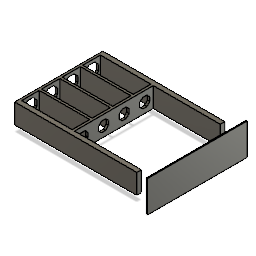
Toolkit Stand v3 (Autodesk Fusion 360 design; units mm, degrees)
Autodesk Fusion 360 part; units mm, degrees
sketch "Sketch1" plane through (0, 0, 0) normal (1, 0, 0) x (0, 0, -1)
  line L0 (0, 0) -> (75, 0)
  line L1 (75, 0) -> (75, 13)
  line L2 (75, 13) -> (0, 13)
  line L3 (0, 13) -> (0, 0)
  line L4 (37.5, 0) -> (37.5, 13)
  line L5 (37.5, 6.5) -> (34.5, 6.5)
  line L6 (37.5, 6.5) -> (40.5, 6.5)
  line L7 (34.5, 6.5) -> (23, 6.5)
  line L8 (34.5, 8.8817) -> (31.1317, 12.25)
  line L9 (31.1317, 12.25) -> (26.3683, 12.25)
  line L10 (26.3683, 12.25) -> (23, 8.8817)
  line L11 (23, 8.8817) -> (23, 4.1183)
  line L12 (23, 4.1183) -> (26.3683, 0.75)
  line L13 (26.3683, 0.75) -> (31.1317, 0.75)
  line L14 (31.1317, 0.75) -> (34.5, 4.1183)
  line L15 (34.5, 4.1183) -> (34.5, 8.8817)
  line L16 (23, 6.5) -> (17, 6.5)
  line L17 (17, 6.5) -> (5.5, 6.5)
  line L18 (5.5, 4.1183) -> (8.8683, 0.75)
  line L19 (8.8683, 0.75) -> (13.6317, 0.75)
  line L20 (13.6317, 0.75) -> (17, 4.1183)
  line L21 (17, 4.1183) -> (17, 8.8817)
  line L22 (17, 8.8817) -> (13.6317, 12.25)
  line L23 (13.6317, 12.25) -> (8.8683, 12.25)
  line L24 (8.8683, 12.25) -> (5.5, 8.8817)
  line L25 (5.5, 8.8817) -> (5.5, 4.1183)
  line L26 (40.5, 6.5) -> (52, 6.5)
  line L27 (40.5, 4.1183) -> (43.8683, 0.75)
  line L28 (43.8683, 0.75) -> (48.6317, 0.75)
  line L29 (48.6317, 0.75) -> (52, 4.1183)
  line L30 (52, 4.1183) -> (52, 8.8817)
  line L31 (52, 8.8817) -> (48.6317, 12.25)
  line L32 (48.6317, 12.25) -> (43.8683, 12.25)
  line L33 (43.8683, 12.25) -> (40.5, 8.8817)
  line L34 (40.5, 8.8817) -> (40.5, 4.1183)
  line L35 (52, 6.5) -> (58, 6.5)
  line L36 (58, 6.5) -> (69.5, 6.5)
  line L37 (58, 4.1183) -> (61.3683, 0.75)
  line L38 (61.3683, 0.75) -> (66.1317, 0.75)
  line L39 (66.1317, 0.75) -> (69.5, 4.1183)
  line L40 (69.5, 4.1183) -> (69.5, 8.8817)
  line L41 (69.5, 8.8817) -> (66.1317, 12.25)
  line L42 (66.1317, 12.25) -> (61.3683, 12.25)
  line L43 (61.3683, 12.25) -> (58, 8.8817)
  line L44 (58, 8.8817) -> (58, 4.1183)
  point P0 (28.75, 6.5)
  point P1 (11.25, 6.5)
  point P2 (46.25, 6.5)
  point P3 (63.75, 6.5)
  dimension "d1" = 75
  dimension "d2" = 13
  dimension "d3" = 3
  dimension "d4" = 3
  dimension "d5" = 11.5
  dimension "d6" = 6
  dimension "d7" = 11.5
  dimension "d8" = 11.5
  dimension "d9" = 6
  dimension "d10" = 11.5
  constraint horizontal L0
  constraint vertical L1
  constraint horizontal L2
  constraint vertical L3
  constraint coincident L0.start L3.end
  constraint midpoint L0 L4.start
  constraint midpoint L2 L4.end
  constraint midpoint L4 L5.start
  constraint perpendicular L4 L5
  constraint perpendicular L4 L6
  constraint parallel L5 L7
  constraint midpoint L7 P0
  constraint perpendicular L11 L16
  constraint parallel L16 L17
  constraint midpoint L17 P1
  constraint parallel L6 L26
  constraint midpoint L26 P2
  constraint perpendicular L30 L35
  constraint parallel L35 L36
  constraint midpoint L36 P3
  measures "d1" distance of L0.start L0.end
  measures "d2" distance of L0.start L2.end
  measures "d3" distance of L5.start L5.end
  measures "d4" distance of L5.start L6.end
  measures "d5" distance of L5.end L7.end
  measures "d6" distance of L7.end L16.end
  measures "d7" distance of L16.end L17.end
  measures "d8" distance of L6.end L26.end
  measures "d9" distance of L26.end L35.end
  measures "d10" distance of L35.end L36.end
extrude "Extrude1" add sketch "Sketch1" along normal blind 2 makes body 1
sketch "Sketch2" plane through (2, 0, 0) normal (1, 0, 0) x (0, 0, -1)
  line L0 (40.5, 4.1183) -> (40.5, 8.8817)
  line L1 (40.5, 8.8817) -> (43.8683, 12.25)
  line L2 (43.8683, 12.25) -> (48.6317, 12.25)
  line L3 (48.6317, 12.25) -> (52, 8.8817)
  line L4 (52, 8.8817) -> (52, 4.1183)
  line L5 (52, 4.1183) -> (48.6317, 0.75)
  line L6 (48.6317, 0.75) -> (43.8683, 0.75)
  line L7 (43.8683, 0.75) -> (40.5, 4.1183)
  line L8 (58, 4.1183) -> (58, 8.8817)
  line L9 (58, 8.8817) -> (61.3683, 12.25)
  line L10 (61.3683, 12.25) -> (66.1317, 12.25)
  line L11 (66.1317, 12.25) -> (69.5, 8.8817)
  line L12 (69.5, 8.8817) -> (69.5, 4.1183)
  line L13 (69.5, 4.1183) -> (66.1317, 0.75)
  line L14 (66.1317, 0.75) -> (61.3683, 0.75)
  line L15 (61.3683, 0.75) -> (58, 4.1183)
  line L16 (5.5, 4.1183) -> (5.5, 8.8817)
  line L17 (5.5, 8.8817) -> (8.8683, 12.25)
  line L18 (8.8683, 12.25) -> (13.6317, 12.25)
  line L19 (13.6317, 12.25) -> (17, 8.8817)
  line L20 (17, 8.8817) -> (17, 4.1183)
  line L21 (17, 4.1183) -> (13.6317, 0.75)
  line L22 (13.6317, 0.75) -> (8.8683, 0.75)
  line L23 (8.8683, 0.75) -> (5.5, 4.1183)
  line L24 (34.5, 8.8817) -> (34.5, 4.1183)
  line L25 (34.5, 4.1183) -> (31.1317, 0.75)
  line L26 (31.1317, 0.75) -> (26.3683, 0.75)
  line L27 (26.3683, 0.75) -> (23, 4.1183)
  line L28 (23, 4.1183) -> (23, 8.8817)
  line L29 (23, 8.8817) -> (26.3683, 12.25)
  line L30 (26.3683, 12.25) -> (31.1317, 12.25)
  line L31 (31.1317, 12.25) -> (34.5, 8.8817)
  line L32 (0, 13) -> (0, 0)
  line L33 (0, 0) -> (75, 0)
  line L34 (75, 0) -> (75, 13)
  line L35 (75, 13) -> (0, 13)
  line L36 (0, 13) -> (2, 13)
  line L37 (2, 13) -> (2, 0)
  line L38 (2, 0) -> (0, 0)
  line L39 (0, 0) -> (0, 13)
  line L40 (75, 0) -> (73, 0)
  line L41 (73, 0) -> (73, 13)
  line L42 (73, 13) -> (75, 13)
  line L43 (75, 13) -> (75, 0)
  dimension "d13" = 2
  dimension "d14" = 2
  constraint horizontal L36
  constraint vertical L37
  constraint horizontal L38
  constraint vertical L39
  constraint coincident L32.start L35.end
  constraint horizontal L40
  constraint vertical L41
  constraint horizontal L42
  constraint vertical L43
  constraint coincident L33.end L34.start
  measures "d13" distance of L32.start L36.end
  measures "d14" distance of L33.end L40.end
extrude "Extrude2" add sketch "Sketch2" along normal blind 45 contours L32 L33 L35 L36 L37 L38 L39 | L33 L34 L35 L40 L41 L42 L43 bodies 1
sketch "Sketch3" plane through (0, 0, -73) normal (0, 0, 1) x (1, 0, 0)
  line L0 (2, 13) -> (2, 0)
  line L1 (2, 0) -> (47, 0)
  line L2 (47, 0) -> (47, 13)
  line L3 (47, 13) -> (2, 13)
  line L4 (47, 13) -> (45, 13)
  line L5 (45, 13) -> (45, 0)
  line L6 (45, 0) -> (47, 0)
  line L7 (47, 0) -> (47, 13)
  dimension "d17" = 2
  constraint horizontal L4
  constraint vertical L5
  constraint horizontal L6
  constraint vertical L7
  constraint coincident L2.end L3.start
  measures "d17" distance of L2.end L4.end
extrude "Extrude3" add sketch "Sketch3" along normal blind 71 contours L1 L2 L3 L4 L5 L6 L7 bodies 1
sketch "Sketch4" plane through (0, 0, 0) normal (-1, 0, 0) x (0, 0, 1)
  line L0 (-40.5, 8.8817) -> (-40.5, 4.1183)
  line L1 (-40.5, 4.1183) -> (-43.8683, 0.75)
  line L2 (-43.8683, 0.75) -> (-48.6317, 0.75)
  line L3 (-48.6317, 0.75) -> (-52, 4.1183)
  line L4 (-52, 4.1183) -> (-52, 8.8817)
  line L5 (-52, 8.8817) -> (-48.6317, 12.25)
  line L6 (-48.6317, 12.25) -> (-43.8683, 12.25)
  line L7 (-43.8683, 12.25) -> (-40.5, 8.8817)
  line L8 (-58, 8.8817) -> (-58, 4.1183)
  line L9 (-58, 4.1183) -> (-61.3683, 0.75)
  line L10 (-61.3683, 0.75) -> (-66.1317, 0.75)
  line L11 (-66.1317, 0.75) -> (-69.5, 4.1183)
  line L12 (-69.5, 4.1183) -> (-69.5, 8.8817)
  line L13 (-69.5, 8.8817) -> (-66.1317, 12.25)
  line L14 (-66.1317, 12.25) -> (-61.3683, 12.25)
  line L15 (-61.3683, 12.25) -> (-58, 8.8817)
  line L16 (-5.5, 8.8817) -> (-5.5, 4.1183)
  line L17 (-5.5, 4.1183) -> (-8.8683, 0.75)
  line L18 (-8.8683, 0.75) -> (-13.6317, 0.75)
  line L19 (-13.6317, 0.75) -> (-17, 4.1183)
  line L20 (-17, 4.1183) -> (-17, 8.8817)
  line L21 (-17, 8.8817) -> (-13.6317, 12.25)
  line L22 (-13.6317, 12.25) -> (-8.8683, 12.25)
  line L23 (-8.8683, 12.25) -> (-5.5, 8.8817)
  line L24 (-34.5, 4.1183) -> (-34.5, 8.8817)
  line L25 (-34.5, 8.8817) -> (-31.1317, 12.25)
  line L26 (-31.1317, 12.25) -> (-26.3683, 12.25)
  line L27 (-26.3683, 12.25) -> (-23, 8.8817)
  line L28 (-23, 8.8817) -> (-23, 4.1183)
  line L29 (-23, 4.1183) -> (-26.3683, 0.75)
  line L30 (-26.3683, 0.75) -> (-31.1317, 0.75)
  line L31 (-31.1317, 0.75) -> (-34.5, 4.1183)
  line L32 (0, 0) -> (0, 13)
  line L33 (0, 13) -> (-75, 13)
  line L34 (-75, 13) -> (-75, 0)
  line L35 (-75, 0) -> (0, 0)
  line L36 (-59.5, 8.2604) -> (-61.9896, 10.75)
  line L37 (-61.9896, 10.75) -> (-65.5104, 10.75)
  line L38 (-65.5104, 10.75) -> (-68, 8.2604)
  line L39 (-68, 8.2604) -> (-68, 4.7396)
  line L40 (-68, 4.7396) -> (-65.5104, 2.25)
  line L41 (-65.5104, 2.25) -> (-61.9896, 2.25)
  line L42 (-61.9896, 2.25) -> (-59.5, 4.7396)
  line L43 (-59.5, 4.7396) -> (-59.5, 8.2604)
  line L44 (-48.0104, 10.75) -> (-50.5, 8.2604)
  line L45 (-50.5, 8.2604) -> (-50.5, 4.7396)
  line L46 (-50.5, 4.7396) -> (-48.0104, 2.25)
  line L47 (-48.0104, 2.25) -> (-44.4896, 2.25)
  line L48 (-44.4896, 2.25) -> (-42, 4.7396)
  line L49 (-42, 4.7396) -> (-42, 8.2604)
  line L50 (-42, 8.2604) -> (-44.4896, 10.75)
  line L51 (-44.4896, 10.75) -> (-48.0104, 10.75)
  line L52 (-24.5, 8.2604) -> (-26.9896, 10.75)
  line L53 (-26.9896, 10.75) -> (-30.5104, 10.75)
  line L54 (-30.5104, 10.75) -> (-33, 8.2604)
  line L55 (-33, 8.2604) -> (-33, 4.7396)
  line L56 (-33, 4.7396) -> (-30.5104, 2.25)
  line L57 (-30.5104, 2.25) -> (-26.9896, 2.25)
  line L58 (-26.9896, 2.25) -> (-24.5, 4.7396)
  line L59 (-24.5, 4.7396) -> (-24.5, 8.2604)
  line L60 (-9.4896, 2.25) -> (-7, 4.7396)
  line L61 (-7, 4.7396) -> (-7, 8.2604)
  line L62 (-7, 8.2604) -> (-9.4896, 10.75)
  line L63 (-9.4896, 10.75) -> (-13.0104, 10.75)
  line L64 (-13.0104, 10.75) -> (-15.5, 8.2604)
  line L65 (-15.5, 8.2604) -> (-15.5, 4.7396)
  line L66 (-15.5, 4.7396) -> (-13.0104, 2.25)
  line L67 (-13.0104, 2.25) -> (-9.4896, 2.25)
  point P0 (-63.75, 6.5)
  point P1 (-46.25, 6.5)
  point P2 (-28.75, 6.5)
  point P3 (-11.25, 6.5)
  dimension "d20" = 4.25
  dimension "d21" = 4.25
  dimension "d22" = 4.25
  dimension "d23" = 4.25
  measures "d20" distance of P0 L43
  measures "d21" distance of P1 L51
  measures "d22" distance of P2 L59
  measures "d23" distance of P3 L67
extrude "Extrude4" cut sketch "Sketch4" against normal blind 80 contours L36 L37 L38 L39 L40 L41 L42 L43 | L44 L45 L46 L47 L48 L49 L50 L51 | L52 L53 L54 L55 L56 L57 L58 L59 | L60 L61 L62 L63 L64 L65 L66 L67 bodies 1
sketch "Sketch5" plane through (47, 0, 0) normal (1, 0, 0) x (0, 0, -1)
  line L0 (24.5, 8.2604) -> (26.9896, 10.75)
  line L1 (26.9896, 10.75) -> (30.5104, 10.75)
  line L2 (30.5104, 10.75) -> (33, 8.2604)
  line L3 (33, 8.2604) -> (33, 4.7396)
  line L4 (33, 4.7396) -> (30.5104, 2.25)
  line L5 (30.5104, 2.25) -> (26.9896, 2.25)
  line L6 (26.9896, 2.25) -> (24.5, 4.7396)
  line L7 (24.5, 4.7396) -> (24.5, 8.2604)
  line L8 (48.0104, 10.75) -> (50.5, 8.2604)
  line L9 (50.5, 8.2604) -> (50.5, 4.7396)
  line L10 (50.5, 4.7396) -> (48.0104, 2.25)
  line L11 (48.0104, 2.25) -> (44.4896, 2.25)
  line L12 (44.4896, 2.25) -> (42, 4.7396)
  line L13 (42, 4.7396) -> (42, 8.2604)
  line L14 (42, 8.2604) -> (44.4896, 10.75)
  line L15 (44.4896, 10.75) -> (48.0104, 10.75)
  line L16 (9.4896, 2.25) -> (7, 4.7396)
  line L17 (7, 4.7396) -> (7, 8.2604)
  line L18 (7, 8.2604) -> (9.4896, 10.75)
  line L19 (9.4896, 10.75) -> (13.0104, 10.75)
  line L20 (13.0104, 10.75) -> (15.5, 8.2604)
  line L21 (15.5, 8.2604) -> (15.5, 4.7396)
  line L22 (15.5, 4.7396) -> (13.0104, 2.25)
  line L23 (13.0104, 2.25) -> (9.4896, 2.25)
  line L24 (59.5, 8.2604) -> (61.9896, 10.75)
  line L25 (61.9896, 10.75) -> (65.5104, 10.75)
  line L26 (65.5104, 10.75) -> (68, 8.2604)
  line L27 (68, 8.2604) -> (68, 4.7396)
  line L28 (68, 4.7396) -> (65.5104, 2.25)
  line L29 (65.5104, 2.25) -> (61.9896, 2.25)
  line L30 (61.9896, 2.25) -> (59.5, 4.7396)
  line L31 (59.5, 4.7396) -> (59.5, 8.2604)
  line L32 (0, 0) -> (75, 0)
  line L33 (75, 0) -> (75, 13)
  line L34 (75, 13) -> (0, 13)
  line L35 (0, 13) -> (0, 0)
  line L36 (75, 0) -> (73, 0)
  line L37 (73, 0) -> (73, 13)
  line L38 (73, 13) -> (75, 13)
  line L39 (75, 13) -> (75, 0)
  line L40 (0, 13) -> (2, 13)
  line L41 (2, 13) -> (2, 0)
  line L42 (2, 0) -> (0, 0)
  line L43 (0, 0) -> (0, 13)
  dimension "d26" = 2
  dimension "d27" = 2
  constraint horizontal L36
  constraint vertical L37
  constraint horizontal L38
  constraint vertical L39
  constraint coincident L32.end L33.start
  constraint horizontal L40
  constraint vertical L41
  constraint horizontal L42
  constraint vertical L43
  constraint coincident L34.end L35.start
  measures "d26" distance of L32.end L36.end
  measures "d27" distance of L34.end L40.end
extrude "Extrude5" add sketch "Sketch5" along normal blind 50 contours L32 L34 L35 L40 L41 L42 L43 | L32 L33 L34 L36 L37 L38 L39 bodies 1
extrude "Extrude6" add 1 faces at (97, 8.6667, -73.6667) along direction (1, 0, 0) blind 3 on bodies 1 bodies 1
extrude "Extrude7" add 1 faces at (97, 8.6667, -0.6667) along direction (1, 0, 0) blind 3 on bodies 1 bodies 1
sketch "Sketch6" plane through (45, 0, 0) normal (-1, 0, 0) x (0, 0, 1)
  line L0 (-26.9896, 10.75) -> (-24.5, 8.2604)
  line L1 (-24.5, 8.2604) -> (-24.5, 4.7396)
  line L2 (-24.5, 4.7396) -> (-26.9896, 2.25)
  line L3 (-26.9896, 2.25) -> (-30.5104, 2.25)
  line L4 (-30.5104, 2.25) -> (-33, 4.7396)
  line L5 (-33, 4.7396) -> (-33, 8.2604)
  line L6 (-33, 8.2604) -> (-30.5104, 10.75)
  line L7 (-30.5104, 10.75) -> (-26.9896, 10.75)
  line L8 (-50.5, 8.2604) -> (-48.0104, 10.75)
  line L9 (-48.0104, 10.75) -> (-44.4896, 10.75)
  line L10 (-44.4896, 10.75) -> (-42, 8.2604)
  line L11 (-42, 8.2604) -> (-42, 4.7396)
  line L12 (-42, 4.7396) -> (-44.4896, 2.25)
  line L13 (-44.4896, 2.25) -> (-48.0104, 2.25)
  line L14 (-48.0104, 2.25) -> (-50.5, 4.7396)
  line L15 (-50.5, 4.7396) -> (-50.5, 8.2604)
  line L16 (-7, 4.7396) -> (-9.4896, 2.25)
  line L17 (-9.4896, 2.25) -> (-13.0104, 2.25)
  line L18 (-13.0104, 2.25) -> (-15.5, 4.7396)
  line L19 (-15.5, 4.7396) -> (-15.5, 8.2604)
  line L20 (-15.5, 8.2604) -> (-13.0104, 10.75)
  line L21 (-13.0104, 10.75) -> (-9.4896, 10.75)
  line L22 (-9.4896, 10.75) -> (-7, 8.2604)
  line L23 (-7, 8.2604) -> (-7, 4.7396)
  line L24 (-61.9896, 10.75) -> (-59.5, 8.2604)
  line L25 (-59.5, 8.2604) -> (-59.5, 4.7396)
  line L26 (-59.5, 4.7396) -> (-61.9896, 2.25)
  line L27 (-61.9896, 2.25) -> (-65.5104, 2.25)
  line L28 (-65.5104, 2.25) -> (-68, 4.7396)
  line L29 (-68, 4.7396) -> (-68, 8.2604)
  line L30 (-68, 8.2604) -> (-65.5104, 10.75)
  line L31 (-65.5104, 10.75) -> (-61.9896, 10.75)
  line L32 (-73, 13) -> (-73, 0)
  line L33 (-73, 0) -> (-2, 0)
  line L34 (-2, 0) -> (-2, 13)
  line L35 (-2, 13) -> (-73, 13)
  line L36 (-59.5, 6.5) -> (-50.5, 6.5)
  line L37 (-42, 6.5) -> (-33, 6.5)
  line L38 (-24.5, 6.5) -> (-15.5, 6.5)
  line L39 (-20, 6.5) -> (-20, 13)
  line L40 (-37.5, 6.5) -> (-37.5, 13)
  line L41 (-55, 6.5) -> (-55, 13)
  line L42 (-55, 13) -> (-54, 13)
  line L43 (-37.5, 13) -> (-36.5, 13)
  line L44 (-36.5, 13) -> (-36.5, 13.0001)
  line L45 (-36.5, 13.0001) -> (-37.5, 13.0001)
  line L46 (-37.5, 13.0001) -> (-37.5, 13)
  line L47 (-20, 13) -> (-19, 13)
  line L48 (-19, 13) -> (-19, 13.0001)
  line L49 (-19, 13.0001) -> (-20, 13.0001)
  line L50 (-20, 13.0001) -> (-20, 13)
  line L51 (-19, 13.0001) -> (-21, 13.0001)
  line L52 (-21, 13.0001) -> (-21, 0)
  line L53 (-21, 0) -> (-19, 0)
  line L54 (-19, 0) -> (-19, 13.0001)
  line L55 (-36.5, 13.0001) -> (-38.5, 13.0001)
  line L56 (-38.5, 13.0001) -> (-38.5, 0)
  line L57 (-38.5, 0) -> (-36.5, 0)
  line L58 (-36.5, 0) -> (-36.5, 13.0001)
  line L59 (-54, 13) -> (-56, 13)
  line L60 (-56, 13) -> (-56, 0)
  line L61 (-56, 0) -> (-54, 0)
  line L62 (-54, 0) -> (-54, 13)
  dimension "d34" = 1
  dimension "d35" = 2
  dimension "d36" = 2
  dimension "d37" = 2
  constraint midpoint L25 L36.start
  constraint midpoint L15 L36.end
  constraint midpoint L11 L37.start
  constraint midpoint L5 L37.end
  constraint midpoint L1 L38.start
  constraint midpoint L19 L38.end
  constraint midpoint L38 L39.start
  constraint coincident L35 L39.end
  constraint perpendicular L35 L39
  constraint midpoint L37 L40.start
  constraint midpoint L35 L40.end
  constraint midpoint L36 L41.start
  constraint coincident L35 L41.end
  constraint perpendicular L35 L41
  constraint coincident L35 L42.end
  constraint horizontal L43
  constraint vertical L44
  constraint horizontal L45
  constraint vertical L46
  constraint horizontal L47
  constraint vertical L48
  constraint horizontal L49
  constraint vertical L50
  constraint horizontal L51
  constraint vertical L52
  constraint horizontal L53
  constraint vertical L54
  constraint horizontal L55
  constraint vertical L56
  constraint horizontal L57
  constraint vertical L58
  constraint horizontal L59
  constraint vertical L60
  constraint horizontal L61
  constraint vertical L62
  measures "d34" distance of L40.end L43.end
  measures "d35" distance of L48.end L51.end
  measures "d36" distance of L44.end L55.end
  measures "d37" distance of L42.end L59.end
extrude "Extrude8" add sketch "Sketch6" along normal blind 45 contours L35 L38 L39 L51 L52 | L33 L38 L52 L53 L54 | L35 L38 L39 L47 L49 L51 L54 | L33 L37 L56 L57 L58 | L35 L37 L40 L43 L45 L55 L58 | L35 L37 L40 L55 L56 | L33 L36 L60 L61 L62 | L35 L36 L41 L42 L59 L62 | L35 L36 L41 L59 L60 bodies 1
sketch "Sketch7" plane through (100, 0, 0) normal (1, 0, 0) x (0, 0, -1)
  line L0 (75, 13) -> (73, 13)
  line L1 (73, 13) -> (73, 0)
  line L2 (73, 0) -> (75, 0)
  line L3 (75, 0) -> (75, 13)
  line L4 (75, 0) -> (0, 0)
  line L5 (0, 0) -> (0, 13)
  line L6 (0, 13) -> (75, 13)
  line L7 (75, 13) -> (75, 0)
  line L8 (0, 13) -> (2, 13)
  line L9 (2, 13) -> (2, 0)
  line L10 (2, 0) -> (0, 0)
  line L11 (0, 0) -> (0, 13)
  line L12 (0, 13) -> (-5, 13)
  line L13 (-5, 13) -> (-5, 18)
  line L14 (-5, 18) -> (0, 18)
  line L15 (0, 18) -> (0, 13)
  line L16 (-5, 18) -> (80, 18)
  line L17 (80, 18) -> (80, -5)
  line L18 (80, -5) -> (-5, -5)
  line L19 (-5, -5) -> (-5, 18)
  dimension "d40" = 5
  dimension "d41" = 5
  dimension "d42" = 85
  dimension "d43" = 23
  constraint horizontal L4
  constraint vertical L5
  constraint horizontal L6
  constraint vertical L7
  constraint coincident L2.end L3.start
  constraint horizontal L8
  constraint vertical L9
  constraint horizontal L10
  constraint vertical L11
  constraint coincident L4 L9.end
  constraint horizontal L12
  constraint vertical L13
  constraint horizontal L14
  constraint vertical L15
  constraint horizontal L16
  constraint vertical L17
  constraint horizontal L18
  constraint vertical L19
  measures "d40" distance of L5.end L14.end
  measures "d41" distance of L5.end L12.end
  measures "d42" distance of L13.end L16.end
  measures "d43" distance of L13.end L18.end
extrude "Extrude9" add sketch "Sketch7" along normal blind 11 and the other way blind -5 separate body contours L12 L15 L16 L17 L18 L19 | L12 L13 L14 L15 L16 L19 | L1 L4 L6 L9 makes body 2
extrude "Extrude10" cut 1 faces at (111, 8.6667, -25.6667) along direction (-1, 0, 0) blind 1 on bodies 2 bodies 2
extrude "Extrude11" add 1 faces at (106.6667, 18, -23.3333) along direction (0, 1, 0) blind 2 on bodies 2 bodies 2
extrude "Extrude12" add 1 faces at (106.6667, -5, -51.6667) along direction (0, -1, 0) blind 2 on bodies 2 bodies 2
sketch "Sketch8" plane through (110, 0, 0) normal (1, 0, 0) x (0, 0, -1)
  line L0 (73, 0) -> (73, 13)
  line L1 (73, 13) -> (75, 13)
  line L2 (75, 13) -> (75, 0)
  line L3 (75, 0) -> (73, 0)
  line L4 (2, 0) -> (0, 0)
  line L5 (0, 0) -> (0, 13)
  line L6 (0, 13) -> (2, 13)
  line L7 (2, 13) -> (2, 0)
  line L8 (80, -7) -> (80, 20)
  line L9 (80, 20) -> (-5, 20)
  line L10 (-5, 20) -> (-5, -7)
  line L11 (-5, -7) -> (80, -7)
extrude "Extrude13" add sketch "Sketch8" against normal blind 2 contours L0 L1 L2 L3 | L4 L5 L6 L7 bodies 2
extrude "Extrude14" add 1 faces at (105, 8.6667, -49.3333) along direction (-1, 0, 0) blind 2 on bodies 2 bodies 2
extrude "Extrude15" cut 1 faces at (106.3333, 4.3333, -75) along direction (0, 0, -1) blind 0.25 on bodies 2 bodies 2
extrude "Extrude16" cut 1 faces at (104.6667, 4.3333, -2) along direction (0, 0, -1) blind 0.25 on bodies 2 bodies 2
extrude "Extrude17" cut 1 faces at (104.6667, 0, -74.5) along direction (0, -1, 0) blind 0.25 on bodies 2 bodies 2
extrude "Extrude18" cut 1 faces at (104.6667, 0, -0.75) along direction (0, -1, 0) blind 0.25 on bodies 2 bodies 2
extrude "Extrude19" cut 1 faces at (104.6667, 8.5833, 0) along direction (0, 0, 1) blind 0.25 on bodies 2 bodies 2
extrude "Extrude20" cut 1 faces at (104.6667, 4.1667, -73) along direction (0, 0, 1) blind 0.25 on bodies 2 bodies 2
extrude "Extrude21" cut 1 faces at (106.3333, 13, -74.4167) along direction (0, 1, 0) blind 0.25 on bodies 2 bodies 2
extrude "Extrude22" cut 1 faces at (104.6667, 13, -1.4167) along direction (0, 1, 0) blind 0.25 on bodies 2 bodies 2
chamfer "Chamfer1" distance 4 angle 45 4 edges at (103, 6.5, 5) (103, -7, -37.5) (103, 20, -37.5) (103, 6.5, -80) on bodies 2
extrude "Extrude23" cut 1 faces at (110, 2, -51.6667) along direction (-1, 0, 0) blind 2 on bodies 2 bodies 2
sketch "Sketch9" plane through (108, 0, 0) normal (1, 0, 0) x (0, 0, -1)
  line L0 (-0.25, 13.25) -> (2.25, 13.25)
  line L1 (2.25, 13.25) -> (2.25, -0.25)
  line L2 (2.25, -0.25) -> (-0.25, -0.25)
  line L3 (-0.25, -0.25) -> (-0.25, 13.25)
  line L4 (72.75, 13.25) -> (75.25, 13.25)
  line L5 (75.25, 13.25) -> (75.25, -0.25)
  line L6 (75.25, -0.25) -> (72.75, -0.25)
  line L7 (72.75, -0.25) -> (72.75, 13.25)
  line L8 (80, -7) -> (80, 20)
  line L9 (80, 20) -> (-5, 20)
  line L10 (-5, 20) -> (-5, -7)
  line L11 (-5, -7) -> (80, -7)
extrude "Extrude24" add sketch "Sketch9" against normal blind 1 contours L0 L1 L2 L3 | L4 L5 L6 L7 bodies 2
move_body "Move1" bodies 2 to x (1, 0, 0) y (0, 1, 0) z (0, 0, 1) at (10, 0, 0)
extrude "Extrude25" add 2 faces at (100, 8.6667, -73.6667) (100, 8.6667, -0.6667) along direction (1, 0, 0) blind 4 on bodies 1 bodies 1
extrude "Extrude26" add 1 faces at (66, 8.6667, -2) along direction (0, 0, -1) blind 2 on bodies 1 bodies 1
extrude "Extrude27" add 1 faces at (66, 4.3333, -73) along direction (0, 0, 1) blind 2 on bodies 1 bodies 1
extrude "Extrude28" cut 1 faces at (115.6667, 8.75, -72.75) along direction (0, 0, 1) blind 2 on bodies 2 bodies 2
extrude "Extrude29" cut 1 faces at (114.3333, 4.25, -2.25) along direction (0, 0, -1) blind 2 on bodies 2 bodies 2
extrude "Extrude30" add 1 faces at (16.3333, 8.6667, -2) along direction (0, 0, -1) blind 2 on bodies 1 bodies 1
extrude "Extrude31" add 1 faces at (16.3333, 4.3333, -73) along direction (0, 0, 1) blind 2 on bodies 1 bodies 1
extrude "Extrude32" add 2 faces at (50.3333, 13, -1.3333) (66, 13, -71.6667) along direction (0, 1, 0) blind 2 on bodies 1 bodies 1
extrude "Extrude33" add 1 faces at (50.3333, 0, -1.3333) along direction (0, -1, 0) blind 2 on bodies 1 bodies 1
extrude "Extrude34" cut 1 faces at (114.3333, 13.25, -2.75) along direction (0, 1, 0) blind 2 on bodies 2 bodies 2
extrude "Extrude35" cut 1 faces at (114.3333, -0.25, -1.25) along direction (0, -1, 0) blind 2 on bodies 2 bodies 2
extrude "Extrude36" cut 1 faces at (115.6667, -0.25, -73.75) along direction (0, -1, 0) blind 2 on bodies 2 bodies 2
extrude "Extrude37" cut 1 faces at (115.6667, 13.25, -73.75) along direction (0, 1, 0) blind 2 on bodies 2 bodies 2
